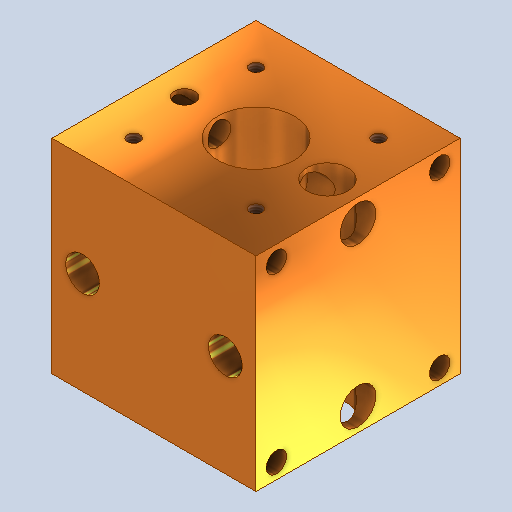
# Autodesk Inventor part: 23
Saved by Autodesk Inventor 2025.1 (Build 291241000, 241)
## iProperties
Created: 2024-09-18
Part Number: 23
Material: Gold
Document SubType Name: Modeling
Designer: ffogue
Density: 19.3 g/cm^3
Appearance: Metal 1600F Hot
Author: ffogue
Autodesk Inventor part; units mm, degrees
note: some values were not read from the file. Chosen so that the rebuilt part matches the saved one: direction of "Hole3"; direction of "Hole4"; direction of "Hole6"; direction of "Hole7"; direction of "Hole1".
ref_plane "YZ Plane" through (0, 0, 0) normal (1, 0, 0) x (0, 1, 0)
ref_plane "XZ Plane" through (0, 0, 0) normal (0, 1, 0) x (-1, 0, 0)
sketch "Sketch1" plane through (0, 0, 0) normal (0, 0, 1) x (1, 0, 0)
  line L0 (-20, -20) -> (20, -20)
  line L1 (20, -20) -> (20, 20)
  line L2 (20, 20) -> (-20, 20)
  line L3 (-20, 20) -> (-20, -20)
  line L4 (-20, -20) -> (20, 20) construction
  line L5 (20, -20) -> (-20, 20) construction
  point P0 (0, 0)
  dimension "d0" = 40
  dimension "d1" = 40
  constraints: 12 end point, 2 midpoint, 2 parallel, 1 horizontal, 1 perpendicular
  measures "d0" distance of L1.end L2.end
  measures "d1" distance of L2.end L0.start
extrude "Extrusion1" add sketch "Sketch1" along normal blind 40
sketch "Sketch2" plane through (0, 0, 40) normal (0, 0, 1) x (1, 0, 0)
  point P0 (0, 0)
  point P1 (0, 0)
  point P2 (-14, 0)
  point P3 (14, 0)
  point P4 (-12, 12)
  point P5 (12, 12)
  point P6 (12, -12)
  point P7 (-12, -12)
  dimension "d5" = 14
  dimension "d6" = 28
  dimension "d7" = 24
  dimension "d8" = 12
  dimension "d9" = 24
  dimension "d10" = 12
  constraints: 4 horizontal alignment, 2 vertical alignment, 1 coincident
  measures "d5" distance of point (0, 0) point (-14, 0)
  measures "d6" distance of point (14, 0) point (-14, 0)
  measures "d7" distance of point (-12, 12) point (-12, -12)
  measures "d8" horizontal distance of point (0, 0) point (-12, -12)
  measures "d9" distance of point (12, 12) point (-12, 12)
  measures "d10" horizontal distance of point (0, 0) point (-12, 12)
hole "Hole2" at (-14, 0, 40) direction (0, 0, -1) diameter 4 depth 15
hole "Hole3" at (-12, 12, 40) at (12, 12, 40) at (12, -12, 40) at (-12, -12, 40) direction (0, 0, -1) diameter 2.459 depth 40 thread size "M3x0.5" class "6H" standard "ISO Metric profile"
hole "Hole4" at (14, 0, 40) direction (0, 0, -1) diameter 8 depth 40
sketch "Sketch3" plane through (20, -20, 0) normal (1, 0, 0) x (0, 0, -1)
  line L0 (0, 40) -> (-40, 40) projected
  line L1 (-40, 0) -> (-40, 40) projected
  line L2 (0, 0) -> (-40, 0) projected
  point P0 (0, 20)
  point P1 (-37, 36)
  point P2 (-3, 36)
  point P3 (-3, 4)
  point P4 (-37, 4)
  point P5 (-35.5, 20)
  point P6 (-4.5, 20)
  point P7 (-40, 20)
  point P8 (-20, 0)
  dimension "d39" = 20
  dimension "d40" = 4.5
  dimension "d41" = 31
  dimension "d42" = 32
  dimension "d43" = 16
  dimension "d44" = 34
  dimension "d45" = 17
  constraints: 3 horizontal alignment, 2 midpoint, 2 vertical alignment
  measures "d39" distance from line of L0 point (-35.5, 20)
  measures "d40" distance from line of L1 point (-35.5, 20)
  measures "d41" distance of point (-4.5, 20) point (-35.5, 20)
  measures "d42" distance of point (-37, 4) point (-37, 36)
  measures "d43" vertical distance of point (-40, 20) point (-37, 36)
  measures "d44" distance of point (-3, 4) point (-37, 4)
  measures "d45" horizontal distance of point (-20, 0) point (-37, 4)
hole "Hole5" at (20, 0, 35.5) at (20, 0, 4.5) direction (-1, 0, 0) diameter 7 depth 20
hole "Hole6" at (20, 16, 37) at (20, 16, 3) at (20, -16, 3) at (20, -16, 37) direction (-1, 0, 0) diameter 4 depth 40
sketch "Sketch4" plane through (-20, 20, 0) normal (0, 1, 0) x (1, 0, 0)
  line L0 (40, 0) -> (40, -40) projected
  line L1 (0, 0) -> (0, -40) projected
  point P0 (20, 0)
  point P1 (6, -20)
  point P2 (34, -20)
  point P3 (0, -20)
  dimension "d60" = 6
  dimension "d61" = 6
  constraints: 2 horizontal alignment, 1 midpoint
  measures "d60" distance from line of L0 point (34, -20)
  measures "d61" distance from line of L1 point (6, -20)
hole "Hole7" at (-14, 20, 20) at (14, 20, 20) direction (0, -1, 0) diameter 6.647 depth 40 thread size "M8x1.25" class "6H" standard "ISO Metric profile"
sketch "Sketch6" plane through (-20, -20, 0) normal (-1, 0, 0) x (0, 0, 1)
  line L0 (0, 40) -> (40, 40) projected
  line L1 (0, 40) -> (0, 0) projected
  point P0 (0, 20)
  point P1 (12, 20)
  point P2 (20, 20)
  point P3 (28, 20)
  point P4 (20, 40)
  point P5 (0, 20)
  dimension "d69" = 16
  dimension "d70" = 8
  constraints: 3 horizontal alignment, 2 midpoint, 1 vertical alignment
  measures "d69" distance of point (28, 20) point (12, 20)
  measures "d70" distance of point (28, 20) point (20, 20)
hole "Hole8" at (-20, 0, 20) direction (1, 0, 0) diameter 6 depth 20
hole "Hole9" at (-20, 0, 12) at (-20, 0, 28) direction (1, 0, 0) diameter 4 depth 20
hole "Hole1" at (0, 0, 40) direction (0, 0, -1) diameter 15 depth 40
sketch "Sketch9" plane through (-20, -20, 0) normal (-1, 0, 0) x (0, 0, 1)
  circle A0 centre (3, 36) radius 2 projected
  circle A1 centre (37, 36) radius 2 projected
  line L0 (0, 40) -> (0, 0) projected
  point P0 (0, 20)
  point P1 (3, 20)
  point P2 (37, 20)
  point P3 (0, 20)
  constraints: 2 horizontal alignment, 2 vertical alignment, 1 midpoint
hole "Hole10" at (-20, 0, 3) at (-20, 0, 37) direction (1, 0, 0) diameter 4.5 depth 15
ref_plane "Work Plane4" through (0, 0, 20) normal (0, 0, 1) x (1, 0, 0)
mirror "Mirror1" about plane through (0, 0, 20) normal (0, 0, 1) of "Hole2"
equation "\"d1\" = d0"
equation "\"d8\" = 0.5 * d7"
equation "\"d9\" = d7"
equation "\"d10\" = 0.5 * d7"
equation "\"d43\" = 0.5 * d42"
equation "\"d45\" = 0.5 * d44"
equation "\"d61\" = d60"
equation "\"d70\" = 0.5 * d69"
body "Solid1"
